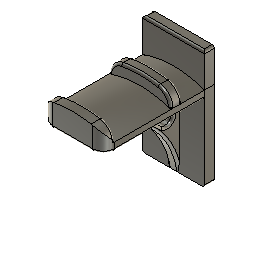
Headphone Mount (Autodesk Fusion 360 design; units mm, degrees)
Autodesk Fusion 360 part; units mm, degrees
sketch "Arm" plane through (0, 0, 0) normal (0, 0, 1) x (1, 0, 0) in component "Mount"
  line L0 (-27.5, 0) -> (27.5, 0)
  line L1 (27.5, 0) -> (27.5, -88.75)
  line L2 (17.5, -98.75) -> (-17.5, -98.75)
  line L3 (-27.5, -88.75) -> (-27.5, 0)
  arc A0 (17.5, -98.75) -> (27.5, -88.75) centre (17.5, -88.75) ccw
  line L4 (0, 0) -> (0, -98.75) construction
  arc A1 (-27.5, -88.75) -> (-17.5, -98.75) centre (-17.5, -88.75) ccw
  line L5 (-5, -8.75) -> (-5, -88.75)
  line L6 (27.5, -88.75) -> (-27.5, -88.75)
  line L7 (27.5, -38.75) -> (-27.5, -38.75)
  line L8 (27.5, -28.75) -> (-27.5, -28.75)
  line L9 (-27.5, -8.75) -> (27.5, -8.75)
  line L10 (-19.05, 0) -> (-19.05, -3.75)
  line L11 (-19.05, -3.75) -> (19.05, -3.75)
  line L12 (19.05, -3.75) -> (19.05, 0)
  line L13 (5, -8.75) -> (5, -88.75)
  circle A2 centre (0, -33.75) radius 1.6
  circle A3 centre (0, -33.75) radius 2.2
  circle A4 centre (0, -33.75) radius 3
  line L14 (5, -8.75) -> (5, -3.75)
  line L15 (-5, -8.75) -> (-5, -3.75)
  point P0 (0, -3.75)
  point P1 (0, -33.75)
  dimension "d1" = 55
  dimension "d5" = 10
  dimension "d7" = 5
  dimension "d8" = 10
  dimension "d12" = 50
  dimension "d13" = 10
  dimension "d15" = 8.75
  dimension "d16" = 20
  dimension "d20" = 3.75
  dimension "d21" = 38.1
  dimension "d23" = 5
  dimension "d24" = 3.2
  dimension "d25" = 4.4
  dimension "d26" = 6
  dimension "d27" = 116.75
  constraint horizontal L0
  constraint vertical L1
  constraint horizontal L2
  constraint vertical L3
  constraint midpoint L0 L4.start
  constraint coincident L4.start origin
  constraint tangent L1 A0
  constraint tangent L2 A0
  constraint coincident L1.end A0.end
  constraint coincident L2.start A0.start
  constraint coincident L2 L4.end
  constraint perpendicular L2 L4
  constraint symmetric L2.start L4 L2.end
  constraint symmetric L1.end L4 L3.start
  constraint symmetric A0 L4 A1
  constraint perpendicular L2 L5
  constraint coincident L1 A0.end
  constraint coincident L3 A1.start
  constraint perpendicular L3 L6
  constraint coincident L1 L7.start
  constraint coincident L3 L7.end
  constraint perpendicular L3 L7
  constraint coincident L1 L8.start
  constraint coincident L3 L8.end
  constraint perpendicular L3 L8
  constraint coincident L3 L9.start
  constraint coincident L1 L9.end
  constraint perpendicular L1 L9
  constraint coincident L9 L5.start
  constraint coincident L0 L10.start
  constraint perpendicular L0 L10
  constraint perpendicular L1 L11
  constraint coincident L0 L12.end
  constraint perpendicular L0 L12
  constraint midpoint L11 P0
  constraint coincident L4 P0
  constraint coincident L6 L5.end
  constraint symmetric L4 L5.start L13.start
  constraint symmetric L4 L5.end L13.end
  constraint coincident L4 P1
  constraint coincident P1 A2.centre
  constraint concentric A3 A4
  constraint coincident L11 L14.end
  constraint perpendicular L11 L14
  constraint coincident L11 L15.end
  constraint perpendicular L11 L15
  measures "d1" distance of L0.start L0.end
  measures "d5" distance of L2 L1.end
  measures "d7" distance of L4 L5
  measures "d8" distance of L2 L6
  measures "d12" distance of L6 L7
  measures "d13" distance of L7 L8
  measures "d15" distance of L0 L9
  measures "d16" distance of L8 L9
  measures "d20" distance of L10.start L10.end
  measures "d21" distance of L10.end L11.end
  measures "d23" distance of L7 P1
  measures "d24" diameter of A2
  measures "d25" diameter of A3
  measures "d26" diameter of A4
extrude "Extrude1" add sketch "Arm" along normal blind 7 contours L3 L5 L8 L9 | L3 L5 L7 L8 | L3 L5 L6 L7 | L1 L8 L9 L13 | L2 A0 A1 L6 | L1 L7 L8 L13 | L1 L6 L7 L13 makes body 1 in component "Mount"
extrude "Extrude2" add sketch "Arm" along normal blind 29.875 from surface at 7 contours L0 L3 L9 L10 L11 L15 | L0 L1 L9 L11 L12 L14 | L9 L11 L14 L15 bodies 1 in component "Mount"
extrude "Extrude4" add sketch "Arm" against normal blind 5 from surface at 36.875 contours L0 L10 L11 L12 bodies 1 in component "Mount"
extrude "Extrude3" add sketch "Arm" along normal blind -68.125 and the other way blind -7 separate body contours L0 L3 L9 L10 L11 L15 | L0 L1 L9 L11 L12 L14 | L9 L11 L14 L15 makes body 2 in component "Mount"
extrude "Extrude5" add sketch "Arm" along normal blind 7 contours L5 L8 L9 L13 | L5 L7 L8 L13 | L5 L6 L7 L13 | A2 | A3 | A4 bodies 2 in component "Mount"
sketch "Arm Arcs" plane through (0, -8.75, 0) normal (0, -1, 0) x (1, 0, 0) in component "Mount"
  line L0 (-27.5, 7) -> (-5, 7)
  line L1 (-5, 7) -> (5, 7)
  line L2 (5, 7) -> (27.5, 7)
  line L3 (27.5, 7) -> (27.5, 36.875)
  line L4 (27.5, 36.875) -> (-27.5, 36.875)
  line L5 (-27.5, 36.875) -> (-27.5, 7)
  line L6 (27.5, -68.125) -> (-27.5, -68.125)
  line L7 (27.5, 7) -> (17.5, 7)
  line L8 (-17.5, 7) -> (17.5, 7)
  line L9 (-17.5, 7) -> (-27.5, 7)
  line L10 (27.5, 7) -> (27.5, 36.875)
  line L11 (-27.5, 7) -> (-27.5, 36.875)
  arc A0 (27.5, 7) -> (-27.5, 7) centre (0, -68.125) ccw
  arc A1 (27.5, 17.5707) -> (-27.5, 17.5707) centre (0, -68.125) ccw
  point P0 (0, -68.125)
  dimension "d47" = 180
  constraint midpoint L6 P0
  constraint coincident P0 A0.centre
  constraint coincident L5 A1.end
  constraint coincident L3 A1.start
  measures "d47" diameter of A1
extrude "Extrude6" add sketch "Arm Arcs" along normal up to surface (90 mm away) contours L0 L1 L2 L7 L8 L9 A0 bodies 1 in component "Mount"
extrude "Extrude7" add sketch "Arm Arcs" along normal blind 10 from surface at 20 contours L3 L5 L10 L11 A0 A1 bodies 1 in component "Mount"
extrude "Extrude8" add 1 faces at (23.9065, -38.75, 11.5597) along direction (0, -1, 0) blind 10 from surface at 50 on bodies 1 bodies 1 in component "Mount"
fillet "Fillet1" radius 13.5 4 edges at (27.5, -33.75, 17.5707) (-27.5, -33.75, 17.5707) (-27.5, -93.75, 17.5707) (27.5, -93.75, 17.5707) on bodies 1 in component "Mount"
extrude "Extrude9" cut 2 faces at (25.5354, -96.7854, 7) (-25.5354, -96.7854, 7) along direction (0, 0, 1) blind 25 on bodies 1 bodies 1 in component "Mount"
fillet "Fillet2" radius 2 7 edges at (-27.5, -4.375, 36.875) (27.5, -48.75, 0) (24.5711, -95.8211, 0) (0, -98.75, 0) (-24.5711, -95.8211, 0) (-27.5, -48.75, 0) (27.5, -4.375, 36.875) on bodies 1 2 in component "Mount"
fillet "Fillet2" radius 2 13 edges at (-27.5, -38.75, 7.0415) (-24.3827, -38.75, 15.7114) (0, -38.75, 21.875) (24.3827, -38.75, 15.7114) (27.5, -38.75, 7.0415) (27.5, -28.75, 7.0415) (24.3827, -28.75, 15.7114) (0, -28.75, 21.875) (-24.3827, -28.75, 15.7114) (-27.5, -28.75, 7.0415) (24.3827, -88.75, 15.7114) (0, -88.75, 21.875) (-24.3827, -88.75, 15.7114) on bodies 1 2 in component "Mount"
fillet "Fillet2" radius 2 1 edges at (0, -8.75, 36.875) on bodies 1 2 in component "Mount"
fillet "Fillet2" radius 2 2 edges at (-27.5, -4.375, -68.125) (27.5, -4.375, -68.125) on bodies 1 2 in component "Mount"
extrude "Extrude10" cut sketch "Arm" along normal blind 6 from surface at 7 contours A2 | A3 bodies 1 in component "Mount"
sketch "Sketch5" plane through (0, 0, 0) normal (1, 0, 0) x (0, 1, 0) in component "Mount"
  line L0 (-8.75, -68.125) -> (-8.75, 0)
  line L1 (-8.75, 0) -> (-88.75, 0)
  arc A0 (-8.75, -68.125) -> (-88.75, 0) centre (-88.75, -81.035) ccw
  line L2 (-37.1664, -13.4721) -> (-23.75, -25.4721)
  arc A1 (-23.75, -25.4721) -> (-15.75, -16.5279) centre (-19.75, -21) ccw
  line L3 (-15.75, -16.5279) -> (-29.1664, -4.5279)
  arc A2 (-29.1664, -4.5279) -> (-37.1664, -13.4721) centre (-33.1664, -9) ccw
  line L4 (-37.6385, -5) -> (-15.2779, -25) construction
  line L5 (0, 0) -> (-88.75, 0) construction
  point P0 (-8.75, -68.125)
  point P1 (-88.75, 0)
  point P2 (-8.75, 0)
  dimension "d65" = 12
  dimension "d66" = 9
  dimension "d67" = 21
  dimension "d68" = 11
  dimension "d69" = 18
  constraint coincident P0 L0.start
  constraint coincident P2 L0.end
  constraint coincident P1 L1.end
  constraint tangent L1 A0
  constraint tangent L2 A1
  constraint tangent A1 L3
  constraint parallel L2 L3
  constraint tangent L3 A2
  constraint tangent L2 A2
  constraint midpoint A2 L4.start
  constraint midpoint A1 L4.end
  measures "d65" distance of L2 L3
  measures "d66" distance of A2.centre L5
  measures "d67" distance of A1.centre L5
  measures "d68" distance of L0 A1.centre
  measures "d69" distance of A2.centre A1.centre
extrude "Extrude11" add sketch "Sketch5" along normal mid plane 10 bodies 2 in component "Mount"
extrude "Extrude12" cut sketch "Arm" along normal blind 7 and the other way blind 39 contours A2 bodies 2 in component "Mount"
extrude "Extrude13" cut sketch "Arm" against normal blind 10 from surface at 2 contours A3 | A4 bodies 2 in component "Mount"
extrude "Extrude14" cut sketch "Arm" along normal blind 7 from surface at 7 contours A2 bodies 1 in component "Mount"
fillet "Fillet4" radius 2 8 edges at (-5, -30.4582, -19.4721) (-5, -15.2779, -25) (-5, -22.4582, -10.5279) (-5, -37.6385, -5) (5, -30.4582, -19.4721) (5, -37.6385, -5) (5, -22.4582, -10.5279) (5, -15.2779, -25) on bodies 2 in component "Mount"
fillet "Fillet4" radius 2 2 edges at (5, -36.2119, -19.3388) (-5, -36.2119, -19.3388) on bodies 2 in component "Mount"
component "Mount" placed x (1, 0, 0) y (0, 1, 0) z (0, 0, 1) at (0, 0, 0)
equation "width = 55 mm"
equation "length = 120 mm"
equation "d5 = split_width"
equation "d8 = split_width"
equation "split_width = 10 mm"
equation "headphone_width = 50 mm"
equation "d12 = headphone_width"
equation "d13 = split_width"
equation "backplate_width = 8.75 mm"
equation "d15 = backplate_width"
equation "d16 = wire_width"
equation "wire_width = 20 mm"
equation "velcro_depth = 3.75 mm"
equation "velcro_width = 38.1 mm"
equation "d20 = velcro_depth"
equation "d21 = velcro_width"
equation "d23 = split_width / 2"
equation "arm_height = 7 mm"
equation "d29 = arm_height"
equation "d31 = back_top_height - arm_height"
equation "d33 = -back_bottom_height"
equation "back_top_height = 36.875 mm"
equation "back_bottom_height = 68.125 mm"
equation "d37 = back_top_height"
equation "d40 = arm_height"
equation "d41 = -arm_height"
equation "d43 = arm_height"
equation "d50 = wire_width"
equation "d51 = split_width"
equation "d53 = headphone_width"
equation "d54 = split_width"
equation "d60 = arm_height"
equation "d73 = arm_height"
named bodies: "Top", "Bottom"
